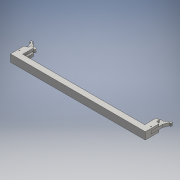
# Autodesk Inventor part: MO-237 10005639-11109LF
Saved by Autodesk Inventor 2016 (Build 200138000, 138)
## iProperties
Created: 2016-07-08
Part Number: MO-237 10005639-11109LF
Material: Generic
Document SubType Name: Modeling
Designer: Jonathan
Density: 1 g/cm^3
Appearance: Default
Author: Jonathan
Autodesk Inventor part; units mm, degrees
ref_plane "YZ Plane" through (0, 0, 0) normal (1, 0, 0) x (0, 1, 0)
ref_plane "XZ Plane" through (0, 0, 0) normal (0, 1, 0) x (-1, 0, 0)
ref_plane "XY Plane" through (0, 0, 0) normal (0, 0, 1) x (1, 0, 0)
sketch "Sketch1" plane through (0, 0, 0) normal (0, 0, 1) x (1, 0, 0)
  line L0 (-70.5, 18.1333) -> (-70.5, 0)
  line L1 (-70.5, 0) -> (70.5, 0)
  line L2 (70.5, 0) -> (70.5, 18.1333)
  line L3 (70.5, 18.1333) -> (63.8333, 18.1333)
  line L4 (63.8333, 18.1333) -> (63.8333, 6)
  line L5 (63.8333, 6) -> (-63.8333, 6)
  line L6 (-63.8333, 6) -> (-63.8333, 18.1333)
  line L7 (-63.8333, 18.1333) -> (-70.5, 18.1333)
  point P0 (0, 0)
  point P1 (0, 0)
  dimension "d0" = 6.6667
  dimension "d1" = 141
  dimension "d2" = 6
  dimension "d3" = 18.1333
  constraints: 16 end point, 5 perpendicular, 1 coincident, 1 collinear, 1 horizontal, 1 midpoint, 1 parallel, 1 point on line, 1 vertical
  measures "d0" distance between parallel lines of L2 L4
  measures "d1" distance of L0.end L1.end
  measures "d2" distance between parallel lines of L1 L5
  measures "d3" distance of L1.end L2.end
extrude "Extrusion1" add sketch "Sketch1" along normal mid plane 7.6
sketch "Sketch2" plane through (70.5, 0, 3.8) normal (1, 0, 0) x (0, 0, -1)
  line L0 (2.3, 15.1333) -> (2.3, 6)
  line L1 (0, 15.1333) -> (2.3, 15.1333)
  line L2 (5.3, 15.1333) -> (5.3, 6)
  line L3 (5.3, 15.1333) -> (7.6, 15.1333)
  line L4 (7.6, 18.1333) -> (0, 18.1333) projected
  line L5 (0, 0) -> (0, 18.1333) projected
  line L6 (7.6, 18.1333) -> (0, 18.1333) projected
  line L7 (0, 0) -> (0, 18.1333) projected
  line L8 (7.6, 0) -> (0, 0) projected
  line L9 (7.6, 18.1333) -> (7.6, 0) projected
  line L10 (7.6, 18.1333) -> (7.6, 0) projected
  line L11 (7.6, 0) -> (0, 0) projected
  line L12 (2.3, 6) -> (5.3, 6)
  line L13 (7.6, 15.1333) -> (7.6, 18.1333)
  line L14 (7.6, 18.1333) -> (0, 18.1333)
  line L15 (0, 15.1333) -> (0, 18.1333)
  point P0 (3.8, 0)
  point P1 (3.8, 6)
  point P2 (3.8, 0)
  dimension "d6" = 3
  dimension "d7" = 3
  dimension "d8" = 6
  constraints: 16 end point, 4 point on line, 2 collinear, 2 midpoint, 2 parallel, 2 perpendicular, 1 horizontal, 1 vertical alignment
  measures "d6" distance between parallel lines of L4 L3
  measures "d7" distance between parallel lines of L0 L2
  measures "d8" distance between parallel lines of L8 L12
extrude "Extrusion2" cut sketch "Sketch2" against normal blind 3.3333 contours L1 L5 L4 L9 L3 L2 L12 L0
sketch "Sketch3" plane through (0, 0, -3.8) normal (0, 0, -1) x (-1, 0, 0)
  line L0 (-70.5, 15.1333) -> (-67.1667, 15.1333) projected
  line L1 (-68, 15.1333) -> (-70.5, 14.1333)
  line L2 (-70.5, 15.1333) -> (-70.5, 6) projected
  line L3 (-70.5, 14.1333) -> (-70.5, 15.1333)
  line L4 (-70.5, 15.1333) -> (-68, 15.1333)
  point P0 (0, 0)
  dimension "d11" = 2.5
  dimension "d12" = 1
  constraints: 6 end point, 2 perpendicular, 2 point on line
  measures "d11" distance of L0.start L1.start
  measures "d12" distance of L1.end L0.start
extrude "Extrusion3" cut sketch "Sketch3" against normal through all
sketch "Sketch4" plane through (0, 0, -3.8) normal (0, 0, -1) x (-1, 0, 0)
  circle A0 centre (-68.8333, 7.6667) radius 0.5
  line L0 (-70.5, 0) -> (-70.5, 14.1333) projected
  line L1 (-70.5, 14.1333) -> (-67.1667, 14.1333) construction
  line L2 (-70.5, 6) -> (-67.1667, 6) projected
  line L3 (-67.1667, 15.1333) -> (-67.1667, 6) projected
  point P0 (0, 0)
  point P1 (-68.8333, 14.1333)
  dimension "d15" = 1
  dimension "d16" = 1.6667
  constraints: 2 end point, 1 centre point, 1 horizontal, 1 midpoint, 1 point on line, 1 vertical alignment
  measures "d15" diameter of A0
  measures "d16" distance from line of L2 A0.centre
extrude "Extrusion4" cut sketch "Sketch4" against normal through all
fillet "Fillet2" radius 1 1 edges at (63.8333, 18.1333, 0)
sketch "Sketch7" plane through (63.8333, 6, -3.8) normal (-1, 0, 0) x (0, 0, 1)
  line L0 (2.8, 12.1333) -> (4.8, 12.1333)
  line L1 (4.8, 12.1333) -> (4.8, -4)
  line L2 (4.8, -4) -> (2.8, -4)
  line L3 (2.8, -4) -> (2.8, 12.1333)
  line L4 (0, 0) -> (7.6, 0) projected
  line L5 (0, 11.1333) -> (7.6, 11.1333) projected
  line L6 (7.6, 12.1333) -> (0, 12.1333) projected
  point P0 (3.8, -6)
  point P1 (3.8, -4)
  point P2 (3.8, 11.1333)
  dimension "d33" = 4
  dimension "d34" = 2
  constraints: 8 end point, 2 midpoint, 2 parallel, 1 collinear, 1 horizontal, 1 perpendicular, 1 vertical alignment
  measures "d33" distance between parallel lines of L2 L4
  measures "d34" distance between parallel lines of L1 L3
extrude "Extrusion7" cut sketch "Sketch7" against normal blind 3.3333
mirror "Mirror2" about plane through (0, 0, 0) normal (1, 0, 0) of "Extrusion2", "Extrusion3", "Extrusion4", "Fillet2", "Extrusion7"
sketch "Sketch5" plane through (0, 0, 0) normal (0, 0, 1) x (1, 0, 0)
  line L0 (70.5, 18.2833) -> (70.5, 6)
  line L1 (70.5, 6) -> (67.1667, 6)
  line L2 (67.1667, 6) -> (67.1667, 18.2833)
  line L3 (70.5, 18.2833) -> (72.5, 23.2833)
  line L4 (72.5, 23.2833) -> (74, 23.2833)
  line L5 (74, 23.2833) -> (74, 25.2833)
  line L6 (74, 25.2833) -> (72, 25.2833)
  line L7 (68, 21.3167) -> (65.35, 21.3167)
  line L8 (67.1667, 18.2833) -> (65.35, 18.2833)
  arc A0 (65.35, 21.3167) -> (65.35, 18.2833) centre (65.35, 19.8) ccw
  line L9 (63.8333, 18.1333) -> (67.1667, 18.1333) projected
  line L10 (70.5, 6) -> (67.1667, 6) projected
  line L11 (67.1667, 15.1333) -> (67.1667, 6) projected
  line L12 (70.5, 14.1333) -> (70.5, 0) projected
  line L13 (63.8333, 6) -> (63.8333, 18.1333) projected
  line L14 (70.5, 0) -> (-70.5, 0) projected
  line L15 (70.5, 0) -> (70.5, 14.1333) projected
  line L16 (70.5, 2) -> (-70.5, 2) construction
  line L17 (-70.5, 0) -> (-70.5, 18.1333) projected
  line L18 (-63.8333, 6) -> (63.8333, 6) projected
  line L19 (72, 25.2833) -> (72, 24.4899)
  line L20 (72, 24.4899) -> (71.4757, 24.4899)
  line L21 (71.4757, 24.4899) -> (71.1058, 23.6965)
  line L22 (71.1058, 23.6965) -> (70.5815, 23.6965)
  line L23 (70.5815, 23.6965) -> (70.2115, 22.9031)
  line L24 (70.2115, 22.9031) -> (69.6873, 22.9031)
  line L25 (69.6873, 22.9031) -> (69.3173, 22.1097)
  line L26 (69.3173, 22.1097) -> (68.7931, 22.1097)
  line L27 (68.7931, 22.1097) -> (68, 21.3167)
  point P0 (0, 0)
  point P1 (68, 15.1333)
  point P2 (-70.5, 14.1333)
  point P3 (66.2583, 18.2833)
  dimension "d19" = 0.15
  dimension "d22" = 4
  dimension "d23" = 17.8
  dimension "d42" = 5
  dimension "d43" = 1.5
  dimension "d44" = 2
  dimension "d45" = 2
  dimension "d46" = 90
  dimension "d49" = 0.7934
  dimension "d50" = 0.7934
  dimension "d51" = 0.7934
  dimension "d52" = 0.7934
  dimension "d53" = 135
  dimension "d54" = 2
  dimension "d55" = 115
  constraints: 38 end point, 9 parallel, 4 horizontal, 4 perpendicular, 3 collinear, 3 tangent, 2 point on circle, 2 point on line, 1 centre point, 1 horizontal alignment, 1 midpoint, 1 vertical, 1 vertical alignment
  measures "d19" distance between parallel lines of L9 L8
  measures "d22" distance between parallel lines of L16 L18
  measures "d23" distance from line of L16 A0.centre
  measures "d42" vertical distance of L0.start L3.end
  measures "d43" distance of L3.end L4.end
  measures "d44" distance of L4.end L5.end
  measures "d45" distance of L5.end L6.end
  measures "d46" angle of L20 L19
  measures "d49" distance of L6.end L19.end
  measures "d50" distance between parallel lines of L20 L22
  measures "d51" distance between parallel lines of L24 L22
  measures "d52" vertical distance of L24.end L25.end
  measures "d53" angle of L7 L27
  measures "d54" horizontal distance of L0.start L3.end
  measures "d55" angle of L22 L21
extrude "Extrusion5" add sketch "Sketch5" against normal up to surface (3 mm away) from surface at 1.5 separate body
fillet "Fillet1" radius 0.5 2 edges at (74, 25.2833, 0) (74, 23.2833, 0)
sketch "Sketch6" plane through (70.5, 6, -1.5) normal (0, 0, -1) x (-1, 0, 0)
  circle A0 centre (1.6667, 1.6667) radius 0.5
  circle A1 centre (1.6667, 1.6667) radius 0.5 projected
  point P0 (70.5, -6)
  constraints: 2 concentric, 1 centre point
extrude "Extrusion6" add sketch "Sketch6" along normal up to surface (2.3 mm away) bodies 2
mirror "Mirror4" about plane through (0, 0, 0) normal (0, 0, 1) of "Extrusion6" bodies 2
mirror "Mirror3" about plane through (0, 0, 0) normal (1, 0, 0) of "Extrusion5", "Fillet1", "Extrusion6", "Mirror4" bodies 2
sketch "Sketch8" plane through (-63.8333, 6, 3.8) normal (0, 1, 0) x (1, 0, 0)
  line L0 (127.6667, 2.8) -> (0, 2.8)
  line L1 (0, 2.8) -> (0, 4.8)
  line L2 (0, 4.8) -> (127.6667, 4.8)
  line L3 (127.6667, 4.8) -> (127.6667, 2.8)
  point P0 (63.8333, 3.8)
  constraints: 8 end point, 3 coincident, 2 parallel, 1 horizontal, 1 perpendicular
extrude "Extrusion8" cut sketch "Sketch8" against normal up to surface (4 mm away) bodies 1
sketch "Sketch9" plane through (0, 0, 0) normal (0, 0, 1) x (1, 0, 0)
  line L0 (67.1667, 2) -> (-67.1667, 2) projected
  line L1 (-3.325, 2) -> (-4.675, 2)
  line L2 (-4.675, 5.125) -> (-4.675, 2)
  line L3 (-3.325, 5.125) -> (-3.325, 2)
  arc A0 (-3.325, 5.125) -> (-4.675, 5.125) centre (-4, 5.125) ccw
  line L4 (-3.5, 5.8) -> (-4.5, 5.8) construction
  point P0 (0, 0)
  point P1 (-4, 5.8)
  dimension "d39" = 1.35
  dimension "d40" = 1
  dimension "d41" = 3.8
  dimension "d57" = 4
  constraints: 8 end point, 3 point on circle, 2 point on line, 2 tangent, 1 centre point, 1 horizontal, 1 midpoint, 1 parallel, 1 perpendicular
  measures "d39" distance between parallel lines of L2 L3
  measures "d40" distance of L4.start L4.end
  measures "d41" distance between parallel lines of L0 L4
  measures "d57" horizontal distance of point (0, 0) A0.centre
extrude "Extrusion9" add sketch "Sketch9" against normal up to surface (2 mm away) from surface at 1 bodies 1
body "Solid1"
body "Solid2"
